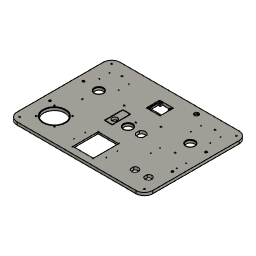
top_plate (Autodesk Fusion 360 design; units mm, degrees)
Autodesk Fusion 360 part; units mm, degrees
sketch "Sketch1" plane through (0, 0, 0) normal (0, 0, 1) x (1, 0, 0)
  line L0 (19, 0) -> (288, 0)
  line L1 (307, 19) -> (307, 214)
  line L2 (288, 233) -> (19, 233)
  line L3 (0, 214) -> (0, 19)
  line L4 (132.25, 72) -> (174.75, 72)
  line L5 (176.75, 70) -> (176.75, 17)
  line L6 (174.75, 15) -> (132.25, 15)
  line L7 (130.25, 17) -> (130.25, 70)
  circle A0 centre (123.5, 116.5) radius 6
  line L8 (114.85, 143.5) -> (132.15, 143.5)
  line L9 (132.15, 143.5) -> (132.15, 102.3)
  line L10 (132.15, 102.3) -> (114.85, 102.3)
  line L11 (114.85, 102.3) -> (114.85, 143.5)
  circle A1 centre (153.5, 116.5) radius 9.55
  circle A2 centre (183.4997, 116.3705) radius 9.6
  line L12 (140, 198) -> (167, 198)
  line L13 (167, 198) -> (167, 179)
  line L14 (167, 179) -> (140, 179)
  line L15 (140, 179) -> (140, 198)
  line L16 (25, 198) -> (75.2, 198)
  line L17 (75.2, 198) -> (75.2, 179)
  line L18 (75.2, 179) -> (25, 179)
  line L19 (25, 179) -> (25, 198)
  line L20 (231.8, 198) -> (282, 198)
  line L21 (282, 198) -> (282, 179)
  line L22 (282, 179) -> (231.8, 179)
  line L23 (231.8, 179) -> (231.8, 198)
  circle A3 centre (50, 53.5) radius 24.25
  circle A4 centre (50.1, 154) radius 9.55
  circle A5 centre (256.9, 154) radius 9.55
  arc A6 (132.25, 72) -> (130.25, 70) centre (132.25, 70) ccw
  arc A7 (176.75, 70) -> (174.75, 72) centre (174.75, 70) ccw
  arc A8 (174.75, 15) -> (176.75, 17) centre (174.75, 17) ccw
  arc A9 (130.25, 17) -> (132.25, 15) centre (132.25, 17) ccw
  arc A10 (19, 233) -> (0, 214) centre (19, 214) ccw
  arc A11 (307, 214) -> (288, 233) centre (288, 214) ccw
  arc A12 (288, 0) -> (307, 19) centre (288, 19) ccw
  arc A13 (0, 19) -> (19, 0) centre (19, 19) ccw
  circle A14 centre (50, 53.5) radius 1.5
  circle A15 centre (276.4, 40) radius 7.65
  circle A16 centre (245.8, 40) radius 7.65
  line L24 (28.1, 200) -> (72.1, 200)
  line L25 (72.1, 200) -> (72.1, 177)
  line L26 (72.1, 177) -> (28.1, 177)
  line L27 (28.1, 177) -> (28.1, 200)
  circle A17 centre (28.1, 200) radius 1
  circle A18 centre (72.1, 200) radius 1
  circle A19 centre (72.1, 177) radius 1
  circle A20 centre (28.1, 177) radius 1
  line L28 (234.9, 200) -> (278.9, 200)
  line L29 (278.9, 200) -> (278.9, 177)
  line L30 (278.9, 177) -> (234.9, 177)
  line L31 (234.9, 177) -> (234.9, 200)
  circle A21 centre (234.9, 200) radius 1
  circle A22 centre (278.9, 200) radius 1
  circle A23 centre (278.9, 177) radius 1
  circle A24 centre (234.9, 177) radius 1
  line L32 (48.5, 208) -> (258.5, 208)
  line L33 (258.5, 208) -> (258.5, 118)
  line L34 (258.5, 118) -> (48.5, 118)
  line L35 (48.5, 118) -> (48.5, 208)
  circle A25 centre (48.5, 208) radius 1.6
  circle A26 centre (258.5, 208) radius 1.6
  circle A27 centre (258.5, 118) radius 1.6
  circle A28 centre (48.5, 118) radius 1.6
  line L36 (232, 110.15) -> (291, 110.15)
  line L37 (291, 110.15) -> (291, 89.65)
  line L38 (291, 89.65) -> (232, 89.65)
  line L39 (232, 89.65) -> (232, 110.15)
  circle A29 centre (291, 110.15) radius 1
  circle A30 centre (232, 110.15) radius 1
  circle A31 centre (232, 89.65) radius 1
  circle A32 centre (291, 89.65) radius 1
  circle A33 centre (114.85, 143.5) radius 1
  circle A34 centre (132.15, 143.5) radius 1
  circle A35 centre (132.15, 102.3) radius 1
  circle A36 centre (114.85, 102.3) radius 1
  circle A37 centre (191.5, 153) radius 1.6
  circle A38 centre (108.5, 153) radius 1.6
  line L40 (138, 203.5) -> (169, 203.5)
  line L41 (169, 203.5) -> (169, 173.5)
  line L42 (169, 173.5) -> (138, 173.5)
  line L43 (138, 173.5) -> (138, 203.5)
  circle A39 centre (141.75, 200.5) radius 1.25
  circle A40 centre (165.25, 200.5) radius 1.25
  circle A41 centre (165.25, 176.5) radius 1.25
  circle A42 centre (141.75, 176.5) radius 1.25
  line L44 (144.9635, 203.5) -> (162.9812, 203.5)
  line L45 (162.9812, 203.5) -> (162.9812, 198)
  line L46 (162.9812, 198) -> (144.9635, 198)
  line L47 (144.9635, 198) -> (144.9635, 203.5)
  circle A43 centre (154.5, 133) radius 1.6
  line L48 (174.9997, 120.8326) -> (174.9997, 111.9085)
  line L49 (191.9997, 120.8326) -> (191.9997, 111.9085)
  line L50 (29.5, 74) -> (70.5, 74)
  line L51 (70.5, 74) -> (70.5, 33)
  line L52 (70.5, 33) -> (29.5, 33)
  line L53 (29.5, 33) -> (29.5, 74)
  circle A44 centre (29.5, 33) radius 1.6
  circle A45 centre (70.5, 33) radius 1.6
  circle A46 centre (70.5, 74) radius 1.6
  circle A47 centre (29.5, 74) radius 1.6
  circle A48 centre (12.5, 12.5) radius 1.6
  circle A49 centre (12.5, 220.5) radius 1.6
  circle A50 centre (294.5, 220.5) radius 1.6
  circle A51 centre (294.5, 12.5) radius 1.6
  line L54 (180.2028, 134.308) -> (188.3229, 134.308) construction
  line L55 (188.3229, 134.308) -> (188.3229, 137.8925) construction
  line L56 (188.3229, 137.8925) -> (180.2028, 137.8925) construction
  line L57 (180.2028, 137.8925) -> (180.2028, 134.308) construction
  line L58 (197.3157, 111.7762) -> (211.2704, 111.7044) construction
  line L59 (211.2704, 111.7044) -> (211.323, 121.9269) construction
  line L60 (211.323, 121.9269) -> (197.3683, 121.9987) construction
  line L61 (197.3683, 121.9987) -> (197.3157, 111.7762) construction
  circle A52 centre (50, 53.5) radius 25.65
  line L62 (130.35, 73.15) -> (176.65, 73.15)
  line L63 (176.65, 73.15) -> (176.65, 13.85)
  line L64 (176.65, 13.85) -> (130.35, 13.85)
  line L65 (130.35, 13.85) -> (130.35, 73.15)
  circle A53 centre (176.65, 73.15) radius 1
  circle A54 centre (130.35, 73.15) radius 1
  circle A55 centre (130.35, 13.85) radius 1
  circle A56 centre (176.65, 13.85) radius 1
  line L66 (127, 81.5) -> (180, 81.5)
  line L67 (180, 81.5) -> (180, 5.5)
  line L68 (180, 5.5) -> (127, 5.5)
  line L69 (127, 5.5) -> (127, 81.5)
  line L70 (190, 56) -> (200, 56)
  line L71 (200, 56) -> (200, 31)
  line L72 (200, 31) -> (190, 31)
  line L73 (190, 31) -> (190, 56)
  line L74 (107, 56) -> (117, 56)
  line L75 (117, 56) -> (117, 31)
  line L76 (117, 31) -> (107, 31)
  line L77 (107, 31) -> (107, 56)
  circle A57 centre (190, 56) radius 1
  circle A58 centre (190, 31) radius 1
  circle A59 centre (117, 31) radius 1
  circle A60 centre (117, 56) radius 1
  line L78 (121.9638, 110.7) -> (125.0362, 110.7)
  line L79 (239.15, 43.7815) -> (239.15, 36.2185)
  line L80 (269.75, 43.7815) -> (269.75, 36.2185)
  circle A61 centre (207, 218) radius 3.2
  circle A62 centre (207, 218) radius 5
  line L81 (292, 154.6) -> (292, 78.4)
  circle A63 centre (292, 78.4) radius 1.85
  circle A64 centre (292, 154.6) radius 1.85
  line L82 (15, 154.6) -> (15, 78.4)
  circle A65 centre (15, 154.6) radius 1.85
  circle A66 centre (15, 78.4) radius 1.85
  circle A67 centre (15, 154.6) radius 2.47
  circle A68 centre (15, 78.4) radius 2.47
  circle A69 centre (292, 78.4) radius 2.47
  circle A70 centre (292, 154.6) radius 2.47
  circle A71 centre (50.1, 154) radius 10.55
  circle A72 centre (256.9, 154) radius 10.55
  circle A73 centre (153.5, 116.5) radius 10.55
  point P0 (307, 0)
  point P1 (0, 233)
  point P2 (130.25, 72)
  point P3 (176.75, 72)
  point P4 (130.25, 15)
  dimension "d3" = 307
  dimension "d4" = 233
  dimension "d21" = 46.5
  dimension "d22" = 57
  dimension "d23" = 130.25
  dimension "d24" = 15
  dimension "d25" = 12
  dimension "d26" = 17.3
  dimension "d27" = 41.2
  dimension "d29" = 27
  dimension "d30" = 8.65
  dimension "d32" = 19.1
  dimension "d33" = 19.2
  dimension "d34" = 153.5
  dimension "d35" = 30
  dimension "d36" = 30
  dimension "d37" = 27
  dimension "d38" = 19
  dimension "d39" = 140
  dimension "d40" = 35
  dimension "d41" = 50.2
  dimension "d42" = 19
  dimension "d43" = 25
  dimension "d44" = 35
  dimension "d45" = 50.2
  dimension "d46" = 19
  dimension "d47" = 25
  dimension "d48" = 35
  dimension "d49" = 48.5
  dimension "d50" = 53.5
  dimension "d51" = 50
  dimension "d52" = 19.1
  dimension "d53" = 25
  dimension "d54" = 50.1
  dimension "d56" = 19.1
  dimension "d57" = 25
  dimension "d58" = 50.1
  dimension "d65" = 2
  dimension "d68" = 19
  dimension "d70" = 3
  dimension "d86" = 15.3
  dimension "d87" = 15.3
  dimension "d88" = 40
  dimension "d89" = 40
  dimension "d90" = 30.6
  dimension "d91" = 30.6
  dimension "d97" = 44
  dimension "d98" = 23
  dimension "d99" = 3.1
  dimension "d100" = 2
  dimension "d101" = 2
  dimension "d102" = 2
  dimension "d103" = 2
  dimension "d104" = 2
  dimension "d105" = 44
  dimension "d106" = 23
  dimension "d107" = 3.1
  dimension "d108" = 2
  dimension "d109" = 2
  dimension "d110" = 2
  dimension "d111" = 2
  dimension "d112" = 2
  dimension "d115" = 90
  dimension "d116" = 210
  dimension "d117" = 91.5
  dimension "d120" = 3.2
  dimension "d121" = 3.2
  dimension "d122" = 3.2
  dimension "d123" = 3.2
  dimension "d126" = 59
  dimension "d127" = 20.5
  dimension "d128" = 16
  dimension "d129" = 49.65
  dimension "d130" = 2
  dimension "d131" = 2
  dimension "d132" = 2
  dimension "d133" = 2
  dimension "d134" = 2
  dimension "d135" = 2
  dimension "d136" = 2
  dimension "d137" = 2
  dimension "d139" = 10
  dimension "d141" = 3.2
  dimension "d142" = 35
  dimension "d143" = 67
  dimension "d144" = 3.2
  dimension "d145" = 35
  dimension "d146" = 150
  dimension "d148" = 116.5
  dimension "d149" = 116.5
  dimension "d157" = 31
  dimension "d158" = 30
  dimension "d159" = 2
  dimension "d160" = 5.5
  dimension "d161" = 2.5
  dimension "d162" = 2.5
  dimension "d163" = 2.5
  dimension "d164" = 2.5
  dimension "d165" = 23.5
  dimension "d166" = 23.5
  dimension "d167" = 24
  dimension "d169" = 24
  dimension "d170" = 2.5
  dimension "d171" = 1.75
  dimension "d172" = 1.75
  dimension "d173" = 2.5
  dimension "d177" = 3.2
  dimension "d178" = 15
  dimension "d179" = 104
  dimension "d180" = 17
  dimension "d181" = 41
  dimension "d182" = 41
  dimension "d183" = 20.5
  dimension "d184" = 20.5
  dimension "d185" = 3.2
  dimension "d186" = 3.2
  dimension "d187" = 3.2
  dimension "d188" = 3.2
  dimension "d190" = 3.2
  dimension "d191" = 12.5
  dimension "d192" = 12.5
  dimension "d193" = 3.2
  dimension "d194" = 12.5
  dimension "d195" = 12.5
  dimension "d196" = 3.2
  dimension "d197" = 12.5
  dimension "d198" = 12.5
  dimension "d199" = 3.2
  dimension "d200" = 12.5
  dimension "d201" = 12.5
  dimension "d203" = 51.3
  dimension "d209" = 46.3
  dimension "d210" = 59.3
  dimension "d212" = 1.15
  dimension "d213" = 0.1
  dimension "d214" = 2
  dimension "d215" = 2
  dimension "d216" = 2
  dimension "d217" = 2
  dimension "d220" = 53
  dimension "d221" = 76
  dimension "d222" = 9.5
  dimension "d223" = 3.25
  dimension "d227" = 10
  dimension "d228" = 25
  dimension "d229" = 10
  dimension "d230" = 25
  dimension "d231" = 25.5
  dimension "d232" = 25.5
  dimension "d234" = 10
  dimension "d235" = 10
  dimension "d236" = 2
  dimension "d237" = 2
  dimension "d238" = 2
  dimension "d239" = 2
  dimension "d241" = 5.8
  dimension "d242" = 6.65
  dimension "d243" = 6.65
  dimension "d247" = 6.4
  dimension "d248" = 10
  dimension "d249" = 15
  dimension "d250" = 100
  dimension "d259" = 76.2
  dimension "d260" = 3.7
  dimension "d261" = 3.7
  dimension "d263" = 15
  dimension "d264" = 78.4
  dimension "d265" = 76.2
  dimension "d266" = 15
  dimension "d267" = 78.4
  dimension "d268" = 3.7
  dimension "d269" = 3.7
  dimension "d272" = 4.94
  dimension "d273" = 4.94
  dimension "d274" = 4.94
  dimension "d275" = 4.94
  dimension "d280" = 21.1
  dimension "d281" = 21.1
  dimension "d282" = 21.1
  constraint horizontal L0
  constraint vertical L1
  constraint horizontal L2
  constraint vertical L3
  constraint horizontal L4
  constraint vertical L5
  constraint horizontal L6
  constraint vertical L7
  constraint horizontal L8
  constraint vertical L9
  constraint horizontal L10
  constraint vertical L11
  constraint horizontal L12
  constraint vertical L13
  constraint horizontal L14
  constraint vertical L15
  constraint horizontal L16
  constraint vertical L17
  constraint horizontal L18
  constraint vertical L19
  constraint horizontal L20
  constraint vertical L21
  constraint horizontal L22
  constraint vertical L23
  constraint coincident P2 L4
  constraint coincident P2 L7
  constraint tangent L4 A6
  constraint tangent L7 A6
  constraint coincident P3 L4
  constraint coincident P3 L5
  constraint tangent L4 A7
  constraint tangent L5 A7
  constraint equal A6 A7
  constraint tangent L5 A8
  constraint tangent L6 A8
  constraint equal A6 A8
  constraint coincident P4 L6
  constraint coincident P4 L7
  constraint tangent L6 A9
  constraint tangent L7 A9
  constraint equal A6 A9
  constraint coincident P1 L2
  constraint coincident P1 L3
  constraint tangent L2 A10
  constraint tangent L3 A10
  constraint tangent L1 A11
  constraint tangent L2 A11
  constraint equal A10 A11
  constraint coincident P0 L0
  constraint coincident P0 L1
  constraint tangent L0 A12
  constraint tangent L1 A12
  constraint equal A10 A12
  constraint coincident origin L0
  constraint coincident origin L3
  constraint tangent L0 A13
  constraint tangent L3 A13
  constraint equal A10 A13
  constraint concentric A3 A14
  constraint horizontal L24
  constraint vertical L25
  constraint horizontal L26
  constraint vertical L27
  constraint coincident L24.start L27.end
  constraint coincident L24.end L25.start
  constraint coincident L25.end L26.start
  constraint coincident L26.end L27.start
  constraint horizontal L28
  constraint vertical L29
  constraint horizontal L30
  constraint vertical L31
  constraint coincident L28.start L31.end
  constraint coincident L28.end L29.start
  constraint coincident L29.end L30.start
  constraint coincident L30.end L31.start
  constraint horizontal L32
  constraint vertical L33
  constraint horizontal L34
  constraint vertical L35
  constraint coincident L32.start L35.end
  constraint coincident L32.end L33.start
  constraint coincident L33.end L34.start
  constraint coincident L34.end L35.start
  constraint horizontal L36
  constraint vertical L37
  constraint horizontal L38
  constraint vertical L39
  constraint coincident L36.end L37.start
  constraint coincident L36.start L39.end
  constraint coincident L38.end L39.start
  constraint coincident L37.end L38.start
  constraint coincident L8.start L11.end
  constraint coincident L8.end L9.start
  constraint coincident L9.end L10.start
  constraint coincident L10.end L11.start
  constraint horizontal L40
  constraint vertical L41
  constraint horizontal L42
  constraint vertical L43
  constraint horizontal L44
  constraint vertical L45
  constraint horizontal L46
  constraint vertical L47
  constraint coincident L12 L45.end
  constraint coincident L40 L44.start
  constraint coincident A2 L48.start
  constraint coincident A2 L48.end
  constraint vertical L48
  constraint coincident A2 L49.start
  constraint coincident A2 L49.end
  constraint vertical L49
  constraint equal L48 L49
  constraint horizontal L50
  constraint vertical L51
  constraint horizontal L52
  constraint vertical L53
  constraint coincident L52.end L53.start
  constraint coincident L51.end L52.start
  constraint coincident L50.end L51.start
  constraint coincident L50.start L53.end
  constraint concentric A14 A52
  constraint horizontal L62
  constraint vertical L63
  constraint horizontal L64
  constraint vertical L65
  constraint coincident L62.end L63.start
  constraint coincident L62.start L65.end
  constraint coincident L64.end L65.start
  constraint coincident L63.end L64.start
  constraint horizontal L66
  constraint vertical L67
  constraint horizontal L68
  constraint vertical L69
  constraint horizontal L70
  constraint vertical L71
  constraint horizontal L72
  constraint vertical L73
  constraint horizontal L74
  constraint vertical L75
  constraint horizontal L76
  constraint vertical L77
  constraint coincident L70.start L73.end
  constraint coincident L72.end L73.start
  constraint coincident L75.end L76.start
  constraint coincident L74.end L75.start
  constraint coincident A0 L78.start
  constraint coincident A0 L78.end
  constraint horizontal L78
  constraint coincident A16 L79.start
  constraint coincident A16 L79.end
  constraint vertical L79
  constraint coincident A15 L80.start
  constraint coincident A15 L80.end
  constraint vertical L80
  constraint concentric A61 A62
  constraint vertical L81
  constraint coincident L81.end A63.centre
  constraint coincident L81.start A64.centre
  constraint vertical L82
  constraint coincident L82.start A65.centre
  constraint coincident L82.end A66.centre
  constraint concentric A64 A70
  constraint concentric A4 A71
  constraint concentric A5 A72
  constraint concentric A1 A73
  measures "d3" distance of origin P0
  measures "d4" distance of origin P1
  measures "d21" distance of P2 P3
  measures "d22" distance of P2 P4
  measures "d23" distance of L3 L7
  measures "d24" distance of L0 L6
  measures "d25" diameter of A0
  measures "d26" distance of L8.start L8.end
  measures "d27" distance of L8.start L10.end
  measures "d29" distance of A0.centre L8
  measures "d30" distance of A0.centre L11
  measures "d32" diameter of A1
  measures "d33" diameter of A2
  measures "d34" distance of L3 A1.centre
  measures "d35" distance of A1.centre A2.centre
  measures "d36" horizontal distance of A0.centre A1.centre
  measures "d37" distance of L12.start L12.end
  measures "d38" distance of L12.start L14.end
  measures "d39" distance of L3 L15
  measures "d40" distance of L2 L12
  measures "d41" distance of L16.start L16.end
  measures "d42" distance of L16.start L18.end
  measures "d43" distance of L3 L19
  measures "d44" distance of L2 L16
  measures "d45" distance of L20.start L20.end
  measures "d46" distance of L20.start L22.end
  measures "d47" distance of L1 L21
  measures "d48" distance of L2 L20
  measures "d49" diameter of A3
  measures "d50" distance of L0 A3.centre
  measures "d51" distance of L3 A3.centre
  measures "d52" diameter of A4
  measures "d53" distance of L18 A4.centre
  measures "d54" distance of L3 A4.centre
  measures "d56" diameter of A5
  measures "d57" distance of L22 A5.centre
  measures "d58" distance of L1 A5.centre
  measures "d65" radius of A6
  measures "d68" radius of A10
  measures "d70" diameter of A14
  measures "d86" diameter of A15
  measures "d87" diameter of A16
  measures "d88" distance of L0 A15.centre
  measures "d89" distance of L0 A16.centre
  measures "d90" distance of A15.centre A16.centre
  measures "d91" distance of L1 A15.centre
  measures "d97" distance of L24.start L24.end
  measures "d98" distance of L24.start L26.end
  measures "d99" distance of L17 L25
  measures "d100" distance of L16 L24
  measures "d101" diameter of A17
  measures "d102" diameter of A18
  measures "d103" diameter of A19
  measures "d104" diameter of A20
  measures "d105" distance of L28.start L28.end
  measures "d106" distance of L28.start L30.end
  measures "d107" distance of L23 L31
  measures "d108" distance of L20 L28
  measures "d109" diameter of A21
  measures "d110" diameter of A22
  measures "d111" diameter of A23
  measures "d112" diameter of A24
  measures "d115" distance of L32.start L34.end
  measures "d116" distance of L33 L35
  measures "d117" distance of L13 L33
  measures "d120" diameter of A25
  measures "d121" diameter of A26
  measures "d122" diameter of A27
  measures "d123" diameter of A28
  measures "d126" distance of L36.start L36.end
  measures "d127" distance of L36.start L38.end
  measures "d128" distance of L1 L37
  measures "d129" distance of A15.centre L38
  measures "d130" diameter of A29
  measures "d131" diameter of A30
  measures "d132" diameter of A31
  measures "d133" diameter of A32
  measures "d134" diameter of A33
  measures "d135" diameter of A34
  measures "d136" diameter of A35
  measures "d137" diameter of A36
  measures "d139" distance of L12 L32
  measures "d141" diameter of A37
  measures "d142" distance of L34 A37.centre
  measures "d143" distance of L33 A37.centre
  measures "d144" diameter of A38
  measures "d145" distance of L34 A38.centre
  measures "d146" distance of L33 A38.centre
  measures "d148" distance of L0 A1.centre
  measures "d149" distance of L0 A0.centre
  measures "d157" distance of L40.start L40.end
  measures "d158" distance of L40.start L42.end
  measures "d159" distance of L15 L43
  measures "d160" distance of L14 L42
  measures "d161" diameter of A39
  measures "d162" diameter of A40
  measures "d163" diameter of A41
  measures "d164" diameter of A42
  measures "d165" distance of A39.centre A40.centre
  measures "d166" horizontal distance of A41.centre A42.centre
  measures "d167" vertical distance of A40.centre A41.centre
  measures "d169" vertical distance of A39.centre A42.centre
  measures "d170" distance of L12 A39.centre
  measures "d171" distance of L13 A41.centre
  measures "d172" distance of L13 A40.centre
  measures "d173" distance of L12 A40.centre
  measures "d177" diameter of A43
  measures "d178" distance of L34 A43.centre
  measures "d179" distance of L33 A43.centre
  measures "d180" distance of L48 L49
  measures "d181" distance of L50.start L50.end
  measures "d182" distance of L50.start L52.end
  measures "d183" distance of A3.centre L53
  measures "d184" distance of A3.centre L50
  measures "d185" diameter of A44
  measures "d186" diameter of A45
  measures "d187" diameter of A46
  measures "d188" diameter of A47
  measures "d190" diameter of A48
  measures "d191" distance of L0 A48.centre
  measures "d192" distance of L3 A48.centre
  measures "d193" diameter of A49
  measures "d194" distance of L3 A49.centre
  measures "d195" distance of L2 A49.centre
  measures "d196" diameter of A50
  measures "d197" distance of L2 A50.centre
  measures "d198" distance of L1 A50.centre
  measures "d199" diameter of A51
  measures "d200" distance of L1 A51.centre
  measures "d201" distance of L0 A51.centre
  measures "d203" diameter of A52
  measures "d209" distance of L62.start L62.end
  measures "d210" distance of L62.start L64.end
  measures "d212" distance of L4 L62
  measures "d213" distance of L5 L63
  measures "d214" diameter of A53
  measures "d215" diameter of A54
  measures "d216" diameter of A55
  measures "d217" diameter of A56
  measures "d220" distance of L66.start L66.end
  measures "d221" distance of L66.start L68.end
  measures "d222" distance of L4 L66
  measures "d223" distance of L7 L69
  measures "d227" distance of L70.start L70.end
  measures "d228" distance of L70.start L72.end
  measures "d229" distance of L74.start L74.end
  measures "d230" distance of L74.start L76.end
  measures "d231" distance of L66 L70
  measures "d232" distance of L66 L74
  measures "d234" distance of L67 L73
  measures "d235" distance of L69 L75
  measures "d236" diameter of A57
  measures "d237" diameter of A58
  measures "d238" diameter of A59
  measures "d239" diameter of A60
  measures "d241" distance of A0.centre L78
  measures "d242" distance of A16.centre L79
  measures "d243" distance of A15.centre L80
  measures "d247" diameter of A61
  measures "d248" diameter of A62
  measures "d249" distance of L2 A61.centre
  measures "d250" distance of L1 A61.centre
  measures "d259" distance of L81.start L81.end
  measures "d260" diameter of A63
  measures "d261" diameter of A64
  measures "d263" distance of L1 L81
  measures "d264" distance of L0 L81.end
  measures "d265" distance of L82.end L82.start
  measures "d266" distance of L3 L82
  measures "d267" distance of L0 L82.end
  measures "d268" diameter of A65
  measures "d269" diameter of A66
  measures "d272" diameter of A67
  measures "d273" diameter of A68
  measures "d274" diameter of A69
  measures "d275" diameter of A70
  measures "d280" diameter of A71
  measures "d281" diameter of A72
  measures "d282" diameter of A73
extrude "Extrude1" add sketch "Sketch1" along normal blind 6.3 contours L0 L1 L2 L3 A10 A11 A12 A13 | L4 A6 A7 L62 L63 L65 A53 A54 | L6 A8 A9 L63 L64 L65 A55 A56 | A0 L78 | A0 L9 L10 L11 L34 A35 A36 | A0 L8 L9 L11 L34 A33 A34 | L8 L9 L11 A2 L16 L17 L18 L20 L22 L23 L24 L25 L26 A18 A19 L28 L30 L31 A21 A24 L32 L33 L34 L35 A25 A26 A27 A28 A33 A34 A71 A72 A73 | L10 L11 A36 | L10 L11 A36 | L8 L11 A33 | L8 L11 A33 | L8 L9 A34 | L8 L9 A34 | L9 L10 A35 | L9 L10 A35 | A1 L34 A73 | A1 L34 A73 | A4 L35 A71 | A4 L35 A71 | A2 L34 L48 | A2 L34 L48 | L18 L25 L26 A19 L35 | L18 L26 L27 A20 L35 | A2 L34 L49 | A2 L34 L49 | L16 L18 L25 L35 | L16 L18 L27 L35 | L16 L17 L18 L25 | L16 L18 L19 L27 | L16 L24 L25 A18 L35 | L16 L24 L27 A17 L35 | A5 L33 A72 | A5 L33 A72 | L22 L29 L30 A23 L33 | L22 L30 L31 A24 L33 | L20 L22 L29 L33 | L20 L22 L31 L33 | L20 L28 L31 A21 L33 | L20 L28 L29 A22 L33 | L20 L21 L22 L29 | L20 L22 L23 L31 | L12 L13 L14 L15 L40 L41 L42 L43 L45 L47 | A3 L51 A52 | A3 L50 L51 A52 | A3 L51 L52 A52 | A3 L50 A52 | L50 L51 A46 A52 | A3 L52 A52 | L51 L52 A45 A52 | A3 L50 L53 A52 | A3 L52 L53 A52 | A3 L53 A52 | L50 L53 A47 A52 | L52 L53 A44 A52 | A15 L80 | A16 L79 | L36 L37 L38 L39 A29 A30 A31 A32 | L37 A29 A32 L81 | L66 L67 L68 L69 | L70 L71 L72 L73 A57 A58 | L74 L75 L76 L77 A59 A60 | A62 | A67 | A68 | A69 | A70 picked at (269.5886, 40.9205) picked at (238.9886, 40.9205)
extrude "Extrude2" cut sketch "Sketch1" against normal blind 0.8 from surface at 6.3 contours A0 L9 L10 L11 L34 A35 A36 | A0 L8 L9 L11 L34 A33 A34 | L10 L11 A36 | L8 L11 A33 | L8 L9 A34 | L9 L10 A35 picked at (115.5133, 102.3474) picked at (115.4998, 143.3587) picked at (131.4867, 143.4526) picked at (132.0087, 102.9498)
extrude "Extrude3" cut sketch "Sketch1" against normal blind 2.5 from surface at 6.3 contours L12 L13 L14 L15 L40 L41 L42 L43 L45 L47 | L12 L40 L44 L45 L46 L47
extrude "Extrude4" cut sketch "Sketch1" against normal blind 0.5 from surface at 6.3 contours A3 L51 A52 | A3 L50 L51 A52 | A3 L51 L52 A52 | A3 L50 A52 | A3 L52 A52 | A3 L50 L53 A52 | A3 L52 L53 A52 | A3 L53 A52
extrude "Extrude5" cut sketch "Sketch1" along normal blind 2.5 contours L4 A6 A7 L62 L63 L65 A53 A54 | L4 L6 A6 A7 A8 A9 L63 L65 | L7 A6 A9 L65 | L5 A7 A8 L63 | L6 A8 A9 L63 L64 L65 A55 A56 | L62 L65 A54 | L62 L65 A54 | L62 L63 A53 | L62 L63 A53 | L64 L65 A55 | L64 L65 A55 | L63 L64 A56 | L63 L64 A56 | L66 L67 L68 L69
extrude "Extrude6" cut sketch "Sketch1" against normal blind 2.5 from surface at 6.3 contours A62
extrude "Extrude7" cut sketch "Sketch1" against normal blind 2 from surface at 6.3 contours A63 | A64 | A65 | A66 | A67 | A68 | A69 | A70
extrude "Extrude8" cut sketch "Sketch1" against normal blind 1.1 from surface at 6.3 contours A1 L34 A73 | A1 L34 A73 | A4 L35 A71 | A4 L35 A71 | A5 L33 A72 | A5 L33 A72
equation "w = 307 mm"
equation "len = 233 mm"
equation "d3 = w"
equation "d4 = len"
equation "key_w = 46.5 mm"
equation "key_l = 57 mm"
equation "led_w = 50.2 mm"
equation "led_l = 19 mm"
equation "btn_d = 19.1 mm"
equation "btn2_d = 19.1 mm"
equation "switch_d = 12 mm"
equation "switch_w = 17.30 mm"
equation "switch_l = 41.2 mm"
equation "switch_hole_offset = 21 mm"
equation "switch_h = 0.8 mm"
equation "oled_w = 27 mm"
equation "oled_l = 19 mm"
equation "keyswitch_d = 19.2 mm"
equation "speaker_d = 48.5 mm"
equation "d21 = key_w"
equation "d22 = key_l"
equation "d23 = ( w - key_w ) / 2"
equation "d25 = switch_d"
equation "d26 = switch_w"
equation "d27 = switch_l"
equation "d29 = switch_hole_offset + switch_d / 2"
equation "d30 = switch_w / 2"
equation "d32 = btn2_d"
equation "d33 = keyswitch_d"
equation "d34 = w / 2"
equation "d37 = screen_x"
equation "d38 = screen_y"
equation "d39 = ( w - oled_w ) / 2"
equation "d40 = led_top_offset + ( led_l - oled_l ) / 2"
equation "d41 = led_w"
equation "d42 = led_l"
equation "d43 = led_offset"
equation "d44 = led_top_offset"
equation "d45 = led_w"
equation "d46 = led_l"
equation "d47 = led_offset"
equation "d48 = led_top_offset"
equation "d49 = speaker_d"
equation "d50 = key_l / 2 + 25 mm"
equation "d52 = btn_d"
equation "d54 = led_w / 2 + led_offset"
equation "led_offset = 25 mm"
equation "d56 = btn_d"
equation "d58 = led_w / 2 + led_offset"
equation "d59 = h"
equation "h = 6.3 mm"
equation "d63 = -switch_h"
equation "d65 = key_f"
equation "key_f = 2 mm"
equation "main_f = 19 mm"
equation "d68 = main_f"
equation "speaker_holes_d = 3 mm"
equation "d70 = speaker_holes_d"
equation "usb_d = 15.3 mm"
equation "d86 = usb_d"
equation "d87 = usb_d"
equation "d90 = usb_d * 2"
equation "d91 = usb_d * 2"
equation "mount_d = 2 mm"
equation "led_m_w = 44 mm"
equation "led_m_l = 23 mm"
equation "d97 = led_m_w"
equation "d98 = led_m_l"
equation "d99 = ( led_w - led_m_w ) / 2"
equation "d100 = ( led_m_l - led_l ) / 2"
equation "d101 = mount_d"
equation "d102 = mount_d"
equation "d103 = mount_d"
equation "d104 = mount_d"
equation "d105 = led_m_w"
equation "d106 = led_m_l"
equation "d107 = ( led_w - led_m_w ) / 2"
equation "d108 = ( led_m_l - led_l ) / 2"
equation "d109 = mount_d"
equation "d110 = mount_d"
equation "d111 = mount_d"
equation "d112 = mount_d"
equation "mainb_m_w = 210 mm"
equation "mainb_m_l = 90 mm"
equation "d115 = mainb_m_l"
equation "d116 = mainb_m_w"
equation "d117 = ( mainb_m_w - oled_w ) / 2"
equation "led_top_offset = 35 mm"
equation "d120 = mount2_d"
equation "d121 = mount2_d"
equation "d122 = mount2_d"
equation "d123 = mount2_d"
equation "charger_w = 59 mm"
equation "charger_l = 20.5 mm"
equation "d126 = charger_w"
equation "d127 = charger_l"
equation "d129 = usb_d / 2 + 42 mm"
equation "d130 = mount_d"
equation "d131 = mount_d"
equation "d132 = mount_d"
equation "d133 = mount_d"
equation "d134 = mount_d"
equation "d135 = mount_d"
equation "d136 = mount_d"
equation "d137 = mount_d"
equation "mount2_d = 3.2 mm"
equation "d141 = mount2_d"
equation "d144 = mount2_d"
equation "middle_offset = len / 2"
equation "d148 = middle_offset"
equation "d149 = middle_offset"
equation "speaker_mount_distance = 41 mm"
equation "screen_b_x = 31 mm"
equation "screen_b_y = 30 mm"
equation "screen_h_x = 23.5 mm"
equation "screen_h_y = 24 mm"
equation "screen_x = 27 mm"
equation "screen_y = 19 mm"
equation "d157 = screen_b_x"
equation "d158 = screen_b_y"
equation "d159 = ( screen_b_x - screen_x ) / 2"
equation "d160 = ( screen_b_y - screen_y ) / 2"
equation "d165 = screen_h_x"
equation "d166 = screen_h_x"
equation "d167 = screen_h_y"
equation "d169 = screen_h_y"
equation "d170 = ( screen_h_y - screen_y ) / 2"
equation "d171 = ( screen_x - screen_h_x ) / 2"
equation "d172 = ( screen_x - screen_h_x ) / 2"
equation "d173 = ( screen_h_y - screen_y ) / 2"
equation "d177 = mount2_d"
equation "d181 = speaker_mount_distance"
equation "d182 = speaker_mount_distance"
equation "d183 = speaker_mount_distance / 2"
equation "d184 = speaker_mount_distance / 2"
equation "d185 = mount2_d"
equation "d186 = mount2_d"
equation "d187 = mount2_d"
equation "d188 = mount2_d"
equation "cmount_distance = 12.50 mm"
equation "d190 = mount2_d"
equation "d191 = cmount_distance"
equation "d192 = cmount_distance"
equation "d193 = mount2_d"
equation "d194 = cmount_distance"
equation "d195 = cmount_distance"
equation "d196 = mount2_d"
equation "d197 = cmount_distance"
equation "d198 = cmount_distance"
equation "d199 = mount2_d"
equation "d200 = cmount_distance"
equation "d201 = cmount_distance"
equation "speaker_grill_d = 51.3 mm"
equation "d203 = speaker_grill_d"
equation "keypad_mount_w = 46.3 mm"
equation "keypad_mount_l = 59.3 mm"
equation "d209 = keypad_mount_w"
equation "d210 = keypad_mount_l"
equation "d212 = ( keypad_mount_l - key_l ) / 2"
equation "d213 = ( key_w - keypad_mount_w ) / 2"
equation "d214 = mount_d"
equation "d215 = mount_d"
equation "d216 = mount_d"
equation "d217 = mount_d"
equation "keypad_platform_w = 53 mm"
equation "keypad_platform_l = 76 mm"
equation "d220 = keypad_platform_w"
equation "d221 = keypad_platform_l"
equation "d222 = ( keypad_platform_l - key_l ) / 2"
equation "d223 = ( keypad_platform_w - key_w ) / 2"
equation "neopixels_mount_distance = 25 mm"
equation "d228 = neopixels_mount_distance"
equation "d230 = neopixels_mount_distance"
equation "d231 = ( keypad_platform_l - neopixels_mount_distance ) / 2"
equation "d232 = ( keypad_platform_l - neopixels_mount_distance ) / 2"
equation "neopixels_offset = 10 mm"
equation "d234 = neopixels_offset"
equation "d235 = neopixels_offset"
equation "d236 = mount_d"
equation "d237 = mount_d"
equation "d238 = mount_d"
equation "d239 = mount_d"
equation "d241 = switch_d / 2 - 0.2 mm"
equation "d242 = usb_d / 2 - 1 mm"
equation "d243 = usb_d / 2 - 1 mm"
equation "antenna_d1 = 6.4 mm"
equation "antenna_d2 = 10 mm"
equation "antenna_h = 2.5 mm"
equation "d247 = antenna_d1"
equation "d248 = antenna_d2"
equation "d252 = -antenna_h"
equation "handle_distance = 76.2 mm"
equation "handle_d = 3.7 mm"
equation "d259 = handle_distance"
equation "d260 = handle_d"
equation "d261 = handle_d"
equation "handle_offset = 15 mm"
equation "d263 = handle_offset"
equation "d264 = ( len - handle_distance ) / 2"
equation "d265 = handle_distance"
equation "d266 = handle_offset"
equation "d267 = ( len - handle_distance ) / 2"
equation "d268 = handle_d"
equation "d269 = handle_d"
equation "handle_d2 = 4.94 mm"
equation "handle_h = 2 mm"
equation "d272 = handle_d2"
equation "d273 = handle_d2"
equation "d274 = handle_d2"
equation "d275 = handle_d2"
equation "d277 = -handle_h"
equation "hole_add = 2 mm"
equation "d280 = btn_d + hole_add"
equation "d281 = btn_d + hole_add"
equation "d282 = btn2_d + hole_add"
equation "hole_add_h = 1.1 mm"
equation "d285 = -hole_add_h"
named bodies: "top_plate"
